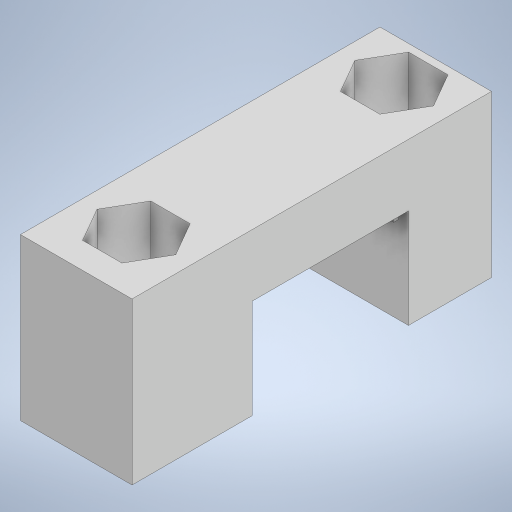
# Autodesk Inventor part: motor_bracket
Saved by Autodesk Inventor 2023 (Build 270158000, 158)
## iProperties
Created: 2024-04-04
Part Number: motor_bracket
Material: Ogólny
Document SubType Name: Modeling
Designer: Kamil
Density: 1 g/cm^3
Appearance: Domyślna
Author: Kamil
Autodesk Inventor part; units mm, degrees
ref_plane "YZ Plane" through (0, 0, 0) normal (1, 0, 0) x (0, 1, 0)
ref_plane "XZ Plane" through (0, 0, 0) normal (0, 1, 0) x (-1, 0, 0)
ref_plane "XY Plane" through (0, 0, 0) normal (0, 0, 1) x (1, 0, 0)
sketch "Szkic1" plane through (0, 0, 0) normal (1, 0, 0) x (0, 1, 0)
  line L0 (-4, 6.3) -> (4, 6.3)
  line L1 (4, 6.3) -> (4, -6.3)
  line L2 (4, -6.3) -> (-4, -6.3)
  line L3 (-4, 6.3) -> (-4, 13)
  line L4 (-4, -6.3) -> (-4, -13)
  line L5 (-1, -13) -> (-1, -9.3)
  line L6 (-1, -9.3) -> (7, -9.3)
  line L7 (7, -9.3) -> (7, 9.3)
  line L8 (7, 9.3) -> (-1, 9.3)
  line L9 (-1, 9.3) -> (-1, 13)
  line L10 (-4, 13) -> (-1, 13)
  line L11 (-4, -13) -> (-1, -13)
  point P0 (0, 0)
  point P1 (0, 6.3)
  point P2 (4, 0)
  dimension "d0" = 8
  dimension "d1" = 12.6
  dimension "d2" = 6.7
  dimension "d3" = 6.7
  dimension "d4" = 3
  constraints: 24 end point, 3 parallel, 2 collinear, 2 horizontal, 2 midpoint, 2 perpendicular, 2 vertical, 1 horizontal alignment, 1 vertical alignment, 4 other
  measures "d0" distance of L1.end L2.end
  measures "d1" distance of L0.end L1.end
  measures "d2" distance of L0.start L3.end
  measures "d3" distance of L2.end L4.end
  measures "d4" distance between parallel lines of L0 L8
extrude "Wyciągnięcie proste1" add sketch "Szkic1" along normal blind 9
sketch "Szkic2" plane through (0, 4, -6.3) normal (0, -1, 0) x (1, 0, 0)
  line L0 (0, 12.6) -> (0, 0) projected
  line L1 (0, 0) -> (9, 0) projected
  line L2 (9, 12.6) -> (9, 0) projected
  line L3 (0, 12.6) -> (9, 12.6) projected
  line L4 (8.2, 12.6) -> (8.2, 0)
  line L5 (4, 12.6) -> (4, 0)
  line L6 (3.2, 12.6) -> (3.2, 0)
  line L7 (0.8, 0) -> (0.8, 12.6)
  line L8 (0.8, 12.6) -> (3.2, 12.6)
  line L9 (3.2, 12.6) -> (3.2, 11.8)
  line L10 (3.2, 11.8) -> (0.8, 11.8)
  line L11 (0.8, 11.8) -> (0.8, 12.6)
  line L12 (0.8, 0) -> (3.2, 0)
  line L13 (3.2, 0) -> (3.2, 0.8)
  line L14 (3.2, 0.8) -> (0.8, 0.8)
  line L15 (0.8, 0.8) -> (0.8, 0)
  line L16 (4, 12.6) -> (8.2, 12.6)
  line L17 (8.2, 12.6) -> (8.2, 11.8)
  line L18 (8.2, 11.8) -> (4, 11.8)
  line L19 (4, 11.8) -> (4, 12.6)
  line L20 (4, 0) -> (8.2, 0)
  line L21 (8.2, 0) -> (8.2, 0.8)
  line L22 (8.2, 0.8) -> (4, 0.8)
  line L23 (4, 0.8) -> (4, 0)
  point P0 (0, 6.3)
  point P1 (4, 0.8)
  point P2 (0.8, 0.8)
  point P3 (0.8, 11.8)
  dimension "d7" = 0.8
  dimension "d8" = 4.2
  dimension "d9" = 0.8
  dimension "d10" = 2.4
  dimension "d11" = 0.8
  dimension "d12" = 0.8
  dimension "d13" = 0.8
  dimension "d14" = 0.8
  constraints: 40 end point, 12 point on line, 8 parallel, 8 perpendicular, 4 horizontal
  measures "d7" distance between parallel lines of L2 L4
  measures "d8" distance between parallel lines of L4 L5
  measures "d9" distance between parallel lines of L5 L6
  measures "d10" distance between parallel lines of L6 L7
  measures "d11" distance between parallel lines of L3 L10
  measures "d12" distance between parallel lines of L1 L14
  measures "d13" distance between parallel lines of L16 L18
  measures "d14" distance between parallel lines of L1 L22
extrude "Wyciągnięcie proste2" add sketch "Szkic2" along normal blind 0.5 contours L3 L6 L10 L7 | L7 L14 L6 L1 | L3 L4 L18 L5 | L5 L22 L4 L1
sketch "Szkic3" plane through (0, 3.5, -6.3) normal (0, -1, 0) x (1, 0, 0)
  line L0 (8.2, 11.8) -> (8.2, 12.6) projected
  line L1 (4, 12.6) -> (8.2, 12.6) projected
  line L2 (4, 12.6) -> (4, 11.8) projected
  line L3 (4, 11.8) -> (8.2, 11.8) projected
  line L4 (3.2, 11.8) -> (3.2, 12.6) projected
  line L5 (0.8, 12.6) -> (3.2, 12.6) projected
  line L6 (0.8, 12.6) -> (0.8, 11.8) projected
  line L7 (0.8, 11.8) -> (3.2, 11.8) projected
  line L8 (0.8, 0.8) -> (0.8, 0) projected
  line L9 (3.2, 0) -> (0.8, 0) projected
  line L10 (3.2, 0) -> (3.2, 0.8) projected
  line L11 (3.2, 0.8) -> (0.8, 0.8) projected
  line L12 (4, 0.8) -> (4, 0) projected
  line L13 (8.2, 0) -> (4, 0) projected
  line L14 (8.2, 0) -> (8.2, 0.8) projected
  line L15 (8.2, 0.8) -> (4, 0.8) projected
  line L16 (8.2, 12.6) -> (8.2, 11.8) projected
  line L17 (8.2, 12.2) -> (0.8, 12.2)
  line L18 (8.2, 0.4) -> (0.8, 0.4)
  point P0 (0, 6.3)
  point P1 (4, 0.4)
  point P2 (3.2, 0.4)
  point P3 (4, 12.2)
  point P4 (3.2, 12.2)
  constraints: 4 end point, 4 midpoint
extrude "Wyciągnięcie proste3" add sketch "Szkic3" along normal blind 0.5 contours L17 L6 L5 L4 | L17 L2 L1 L0 | L18 L14 L13 L12 | L18 L10 L9 L8
sketch "Szkic4" plane through (9, 0, 0) normal (1, 0, 0) x (0, 0, -1)
  line L0 (-6.3, -4) -> (-6.3, 4) projected
  line L1 (-6.3, 4) -> (6.3, 4) projected
  line L2 (6.3, 4) -> (6.3, -4) projected
  line L3 (6.3, -4) -> (13, -4) projected
  line L4 (13, -4) -> (13, -1) projected
  line L5 (13, -1) -> (9.3, -1) projected
  line L6 (9.3, -1) -> (9.3, 7) projected
  line L7 (9.3, 7) -> (-9.3, 7) projected
  line L8 (-9.3, 7) -> (-9.3, -1) projected
  line L9 (-9.3, -1) -> (-13, -1) projected
  line L10 (-13, -1) -> (-13, -4) projected
  line L11 (-13, -4) -> (-6.3, -4) projected
  line L12 (-13, -1) -> (13, -1)
  line L13 (13, -1) -> (13, 9)
  line L14 (13, 9) -> (-13, 9)
  line L15 (-13, 9) -> (-13, -1)
  point P0 (0, 0)
  dimension "d19" = 10
  constraints: 8 end point, 2 parallel, 1 horizontal, 1 perpendicular
  measures "d19" distance of L12.end L13.end
extrude "Wyciągnięcie proste4" add sketch "Szkic4" against normal up to surface (9 mm away) contours L9 L15 L14 L13 L5 L6 L7 L8
sketch "Szkic5" plane through (0, -4, 13) normal (0, 0, 1) x (1, 0, 0)
  line L0 (0, 0) -> (0, 13) projected
  line L1 (0, 0) -> (9, 0) projected
  line L2 (9, 13) -> (9, 0) projected
  line L3 (9, 13) -> (0, 13) projected
  point P0 (0, 4)
extrude "Wyciągnięcie proste5" add sketch "Szkic5" along normal blind 3
sketch "Szkic6" plane through (0, -4, -13) normal (0, -1, 0) x (1, 0, 0)
  line L0 (0, 0) -> (9, 0) projected
  line L1 (0, 6.7) -> (9, 6.7) projected
  line L2 (0, 19.3) -> (9, 19.3) projected
  line L3 (0, 29) -> (9, 29) projected
  line L4 (4.5, 0) -> (4.5, 6.7) construction
  line L5 (4.5, 19.3) -> (4.5, 29) construction
  point P0 (0, 13)
  point P1 (4.5, 3.35)
  point P2 (4.5, 24.15)
  constraints: 6 midpoint, 4 end point
hole "Otwór1" at (4.5, -4, -9.65) at (4.5, -4, 11.15) direction (0, 1, 0) diameter 3.5 depth 8 counterbore diameter 3.9 counterbore depth 4
sketch "Szkic7" plane through (0, 9, -13) normal (0, 1, 0) x (1, 0, 0)
  circle A0 centre (4.5, -3.35) radius 1.75 projected
  circle A1 centre (4.5, -24.15) radius 1.75 projected
  circle A2 centre (4.5, -3.35) radius 2.75
  circle A3 centre (4.5, -24.15) radius 2.75
  line L0 (6.0877, -0.6) -> (7.6754, -3.35)
  line L1 (7.6754, -3.35) -> (6.0877, -6.1)
  line L2 (6.0877, -6.1) -> (2.9123, -6.1)
  line L3 (2.9123, -6.1) -> (1.3246, -3.35)
  line L4 (1.3246, -3.35) -> (2.9123, -0.6)
  line L5 (2.9123, -0.6) -> (6.0877, -0.6)
  line L6 (2.9123, -26.9) -> (1.3246, -24.15)
  line L7 (1.3246, -24.15) -> (2.9123, -21.4)
  line L8 (2.9123, -21.4) -> (6.0877, -21.4)
  line L9 (6.0877, -21.4) -> (7.6754, -24.15)
  line L10 (7.6754, -24.15) -> (6.0877, -26.9)
  line L11 (6.0877, -26.9) -> (2.9123, -26.9)
  point P0 (0, -13)
  point P1 (4.5, -0.6)
  point P2 (4.5, -26.9)
  dimension "d31" = 5.5
  dimension "d32" = 5.5
  constraints: 24 end point, 4 coincident, 2 midpoint, 2 vertical alignment, 30 other
extrude "Wyciągnięcie proste6" cut sketch "Szkic7" against normal blind 5 contours A0 | A1 | A2 | A2 L0 L1 | A2 L5 L0 | L1 L2 A2 | A2 L4 L5 | L2 L3 A2 | A2 L3 L4 | A3 | A3 L9 L10 | A3 L8 L9 | L10 L11 A3 | A3 L7 L8 | L11 L6 A3 | A3 L6 L7
